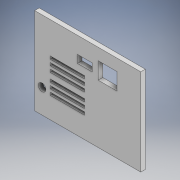
# Autodesk Inventor part: compnent box front
Saved by Autodesk Inventor 2021 (Build 250183000, 183)
## iProperties
Created: 2023-04-24
Part Number: compnent box front
Material: Generic
Document SubType Name: Modeling
Designer: boyle
Density: 1 g/cm^3
Appearance: Default
Author: boyle
Autodesk Inventor part; units mm, degrees
ref_plane "YZ Plane" through (0, 0, 0) normal (1, 0, 0) x (0, 1, 0)
ref_plane "XZ Plane" through (0, 0, 0) normal (0, 1, 0) x (-1, 0, 0)
ref_plane "XY Plane" through (0, 0, 0) normal (0, 0, 1) x (1, 0, 0)
sketch "Sketch1" plane through (0, 0, 0) normal (0, 0, 1) x (1, 0, 0)
  line L0 (0, 0) -> (111.76, 0)
  line L1 (111.76, 0) -> (111.76, 91.44)
  line L2 (111.76, 91.44) -> (0, 91.44)
  line L3 (0, 91.44) -> (0, 0)
  dimension "d0" = 111.76
  dimension "d1" = 91.44
  constraints: 8 end point, 2 parallel, 1 horizontal, 1 perpendicular
  measures "d0" distance of L2.end L1.end
  measures "d1" distance of L1.end L0.end
extrude "Extrusion1" add sketch "Sketch1" along normal blind 4.826
sketch "Sketch2" plane through (0, 0, 4.826) normal (0, 0, 1) x (1, 0, 0)
  line L0 (111.76, 0) -> (111.76, 91.44) projected
  line L1 (34.5493, 37.338) -> (52.5493, 37.338)
  line L2 (52.5493, 40.338) -> (16.5493, 40.338)
  line L3 (16.5493, 43.338) -> (52.5493, 43.338)
  line L4 (34.5493, 46.338) -> (52.5493, 46.338)
  line L5 (16.5493, 49.338) -> (52.5493, 49.338)
  line L6 (52.5493, 52.338) -> (16.5493, 52.338)
  line L7 (34.5493, 55.338) -> (52.5493, 55.338)
  line L8 (16.5493, 58.338) -> (52.5493, 58.338)
  line L9 (16.5493, 58.338) -> (16.5493, 22.338)
  line L10 (52.5493, 22.338) -> (16.5493, 22.338)
  line L11 (34.5493, 25.338) -> (52.5493, 25.338)
  line L12 (34.5493, 28.338) -> (52.5493, 28.338)
  line L13 (34.5493, 31.338) -> (52.5493, 31.338)
  line L14 (34.5493, 34.338) -> (52.5493, 34.338)
  line L15 (66.96, 79.167) -> (86.76, 79.167)
  line L16 (66.96, 61.44) -> (66.96, 79.167)
  line L17 (86.76, 61.44) -> (66.96, 61.44)
  line L18 (86.76, 79.167) -> (86.76, 61.44)
  line L19 (60.6088, 74.0565) -> (60.6088, 65.8015)
  line L20 (60.6088, 65.8015) -> (45.0584, 65.8015)
  line L21 (45.0584, 65.8015) -> (45.0584, 74.0565)
  line L22 (45.0584, 74.0565) -> (60.6088, 74.0565)
  circle A0 centre (7.874, 25.4) radius 4.0005
  line L23 (66.96, 79.167) -> (86.76, 79.167)
  line L24 (86.76, 79.167) -> (86.76, 61.44)
  line L25 (86.76, 61.44) -> (66.96, 61.44)
  line L26 (66.96, 61.44) -> (66.96, 79.167)
  line L27 (52.5493, 58.338) -> (16.5493, 58.338)
  line L28 (16.5493, 58.338) -> (16.5493, 22.338)
  line L29 (16.5493, 22.338) -> (52.5493, 22.338)
  line L30 (52.5493, 22.338) -> (52.5493, 58.338)
  circle A1 centre (7.874, 25.4) radius 4.0005
  line L31 (34.5493, 58.338) -> (34.5493, 22.338)
  line L32 (16.5493, 55.338) -> (52.5493, 55.338)
  line L33 (52.5493, 52.338) -> (16.5493, 52.338)
  line L34 (16.5493, 49.338) -> (52.5493, 49.338)
  line L35 (52.5493, 46.338) -> (16.5493, 46.338)
  line L36 (16.5493, 43.338) -> (52.5493, 43.338)
  line L37 (52.5493, 40.338) -> (16.5493, 40.338)
  line L38 (16.5493, 37.338) -> (52.5493, 37.338)
  line L39 (52.5493, 34.338) -> (16.5493, 34.338)
  line L40 (16.5493, 31.338) -> (52.5493, 31.338)
  line L41 (52.5493, 28.338) -> (16.5493, 28.338)
  line L42 (16.5493, 25.338) -> (52.5493, 25.338)
  line L43 (60.6088, 0) -> (60.6088, 50.8)
  line L44 (111.76, 91.44) -> (111.76, 61.44)
  line L45 (111.76, 61.44) -> (86.76, 61.44)
  line L46 (86.76, 79.167) -> (86.76, 61.44)
  point P0 (0, 0)
  point P1 (0, 0)
  point P2 (0, 0)
  point P3 (0, 0)
  point P4 (0, 0)
  point P5 (16.5493, 28.338)
  dimension "d4" = 50.8
  dimension "d7" = 30
  dimension "d8" = 25
  constraints: 90 end point, 5 collinear, 5 horizontal, 5 parallel, 4 perpendicular, 2 centre point, 2 coincident, 2 midpoint, 2 vertical, 1 concentric, 1 point on line, 10 other
  measures "d4" distance of L43.start L43.end
  measures "d7" distance of L0.end L44.end
  measures "d8" distance of L44.end L45.end
extrude "Extrusion2" cut sketch "Sketch2" against normal blind 4.826 contours L1 L30 L14 L31 | L31 L39 L9 L38 | L13 L30 L12 L31 | L31 L41 L9 L40 | L31 L4 L30 L3 | L3 L9 L35 L31 | L11 L30 L10 L31 | L31 L10 L9 L42 | L31 L6 L30 L5 | L5 L9 L6 L31 | L31 L8 L30 L7 | L32 L9 L8 L31 | L15 L18 L17 L16 | L19 L20 L21 L22 | A0
body "Solid1"
